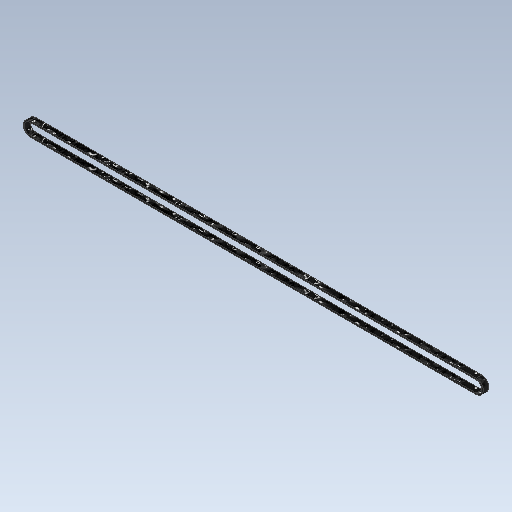
# Autodesk Inventor part: xy-belt
Saved by Autodesk Inventor 2020.4 (Build 244396000, 396)
## iProperties
Created: 2021-03-31
Part Number: xy-belt
Material: Nylon 6/6
Document SubType Name: Modeling
Designer: AOB
Mass: 9.40908 g
Surface Area: 146.707 cm^2
Volume: 8.32662 cm^3
Density: 1.13 g/cm^3
Appearance: Black
Author: AOB
Autodesk Inventor part; units mm, degrees
ref_plane "YZ Plane" through (0, 0, 0) normal (1, 0, 0) x (0, 1, 0)
ref_plane "XZ Plane" through (0, 0, 0) normal (0, 1, 0) x (-1, 0, 0)
ref_plane "XY Plane" through (0, 0, 0) normal (0, 0, 1) x (1, 0, 0)
sketch "Sketch1" plane through (0, 0, 0) normal (0, 0, 1) x (1, 0, 0)
  arc A0 (0, 6.11) -> (0, -6.11) centre (0, 0) ccw
  line L0 (0, 0) -> (474.2377, 0) construction
  arc A1 (474.2377, -6.11) -> (474.2377, 6.11) centre (474.2377, 0) ccw
  line L1 (0, 6.11) -> (474.2377, 6.11)
  line L2 (474.2377, -6.11) -> (0, -6.11)
  arc A2 (0, 7.51) -> (0, -7.51) centre (0, 0) ccw
  arc A3 (474.2377, -7.51) -> (474.2377, 7.51) centre (474.2377, 0) ccw
  line L3 (474.2377, 7.51) -> (0, 7.51)
  line L4 (0, -7.51) -> (474.2377, -7.51)
  dimension "d0" = 12.22
  dimension "d1" = 12.22
  dimension "d2" = 474.2377
  dimension "d3" = 15.02
  dimension "d4" = 15.02
  constraints: 10 end point, 8 point on circle, 4 centre point, 4 coincident, 4 tangent, 2 horizontal, 1 parallel
  measures "d0" diameter of A0
  measures "d1" diameter of A1
  measures "d2" distance of L0.start L0.end
  measures "d3" diameter of A2
  measures "d4" diameter of A3
extrude "Extrusion1" add sketch "Sketch1" along normal blind 6
body "Solid1"
